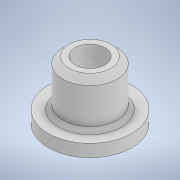
# Autodesk Inventor part: plastic_axis_washer
Saved by Autodesk Inventor 2020 (Build 240168000, 168)
## iProperties
Created: 2020-01-24
Part Number: plastic_axis_washer
Material: Generic
Document SubType Name: Modeling
Designer: erwin
Density: 1 g/cm^3
Appearance: Default
Author: erwin
Autodesk Inventor part; units mm, degrees
ref_plane "YZ Plane" through (0, 0, 0) normal (1, 0, 0) x (0, 1, 0)
ref_plane "XZ Plane" through (0, 0, 0) normal (0, 1, 0) x (-1, 0, 0)
ref_plane "XY Plane" through (0, 0, 0) normal (0, 0, 1) x (1, 0, 0)
sketch "Sketch1" plane through (0, 0, 0) normal (0, 1, 0) x (-1, 0, 0)
  circle A0 centre (0, 0) radius 5
  dimension "d0" = 10
  constraints: 1 centre point, 1 coincident
  measures "d0" diameter of A0
extrude "Extrusion1" add sketch "Sketch1" along normal blind 1
sketch "Sketch2" plane through (0, 1, 0) normal (0, 1, 0) x (1, 0, 0)
  circle A0 centre (0, 0) radius 3.25
  dimension "d3" = 6.5
  constraints: 1 centre point, 1 coincident
  measures "d3" diameter of A0
extrude "Extrusion2" add sketch "Sketch2" along normal blind 5.5
sketch "Sketch3" plane through (0, 6.5, 0) normal (0, 1, 0) x (1, 0, 0)
  circle A0 centre (0, 0) radius 3.25 projected
  constraints: 1 coincident
hole "Hole1" at (0, 6.5, 0) direction (0, -1, 0) diameter 3.6 end through all
chamfer "Chamfer1" distance 0.5 angle 45 2 edges at (-3.25, 6.5, 0) (-3.25, 1, 0)
thicken "Thicken1" operation add thickness 0.5 both sides no extend neighbours yes toward (0, -1, 0) faces at (-3.8805, 0, -0.4712)
chamfer "Chamfer2" distance 1.5 angle 45 1 edges at (0, -0.5, -1.8)
move faces "Move1" translate (0, -0.25, 0) faces at (-1.3863, 6.0833, -2.8471)
body "Solid1"
